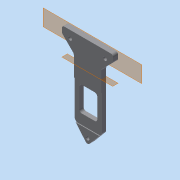
# Autodesk Inventor part: cellSTORM_inverted_chiptray_v0
Saved by Autodesk Inventor 2019.4 (Build 234330000, 330)
## iProperties
Created: 2020-11-09
Part Number: cellSTORM_inverted_chiptray_v0
Material: Generic
Document SubType Name: Modeling
Designer: diederichbenedict
Density: 1 g/cm^3
Appearance: Default
Author: diederichbenedict
Autodesk Inventor part; units mm, degrees
ref_plane "YZ Plane" through (0, 0, 0) normal (1, 0, 0) x (0, 1, 0)
ref_plane "XZ Plane" through (0, 0, 0) normal (0, 1, 0) x (-1, 0, 0)
ref_plane "XY Plane" through (0, 0, 0) normal (0, 0, 1) x (1, 0, 0)
ref_plane "Work Plane1" through (0, 0, 0) normal (0, 0, 1) x (1, 0, 0)
sketch "Sketch1" plane through (0, 0, 0) normal (0, 0, 1) x (1, 0, 0)
  circle A0 centre (-18, 0) radius 2.45 construction
  circle A1 centre (-32.0354, 0) radius 2.45 construction
  circle A2 centre (-48, 0) radius 3.05 construction
  line L0 (18, 6) -> (-54, 6) construction
  line L1 (-54, -6) -> (-54, 6) construction
  line L2 (-54, -6) -> (18, -6) construction
  line L3 (18, -6) -> (18, 6) construction
  circle A3 centre (12, 0) radius 3.05 construction
  circle A4 centre (-3.9646, 0) radius 2.45 construction
  circle A5 centre (-18, -62.5107) radius 2.45 construction
  circle A6 centre (-3.9646, -62.1646) radius 2.45 construction
  circle A7 centre (12, -70) radius 3.05 construction
  line L4 (-32.0354, -67.7344) -> (-3.9646, -67.7344) construction
  line L5 (-3.9646, -67.7344) -> (14.2856, -76.6915) construction
  line L6 (14.2856, -76.6915) -> (18.6915, -67.7144) construction
  line L7 (18.6915, -67.7144) -> (-2.5545, -57.2869) construction
  line L8 (-33.4455, -57.2869) -> (-2.5545, -57.2869) construction
  line L9 (-54.6915, -67.7144) -> (-33.4455, -57.2869) construction
  line L10 (-50.2856, -76.6915) -> (-54.6915, -67.7144) construction
  line L11 (-32.0354, -67.7344) -> (-50.2856, -76.6915) construction
  circle A8 centre (-48, -70) radius 3.05 construction
  circle A9 centre (-32.0354, -62.1646) radius 2.45 construction
  line L12 (-30, -24.7225) -> (-6, -24.7225) construction
  line L13 (-6, -24.7225) -> (-6, -18.4525) construction
  line L14 (-6, -18.4525) -> (-30, -18.4525) construction
  line L15 (-30, -18.4525) -> (-30, -24.7225) construction
  line L16 (-6, -33.7225) -> (-11.7463, -33.7225) construction
  line L17 (-6, -33.34) -> (-6, -33.7225) construction
  line L18 (-6, -33.34) -> (-11.7042, -33.34) construction
  line L19 (-6, -32.95) -> (-6, -33.34) construction
  line L20 (-6, -32.95) -> (-11.6853, -32.95) construction
  line L21 (-6, -32.56) -> (-6, -32.95) construction
  line L22 (-6, -32.56) -> (-11.6906, -32.56) construction
  line L23 (-6, -32.17) -> (-6, -32.56) construction
  line L24 (-6, -32.17) -> (-11.72, -32.17) construction
  line L25 (-6, -31.78) -> (-6, -32.17) construction
  line L26 (-6, -31.78) -> (-11.7739, -31.78) construction
  line L27 (-6, -31.39) -> (-6, -31.78) construction
  line L28 (-6, -31.39) -> (-11.8531, -31.39) construction
  line L29 (-6, -31) -> (-6, -31.39) construction
  line L30 (-6, -31) -> (-11.9583, -31) construction
  line L31 (-6, -30.61) -> (-6, -31) construction
  line L32 (-6, -30.61) -> (-12.0912, -30.61) construction
  line L33 (-6, -30.22) -> (-6, -30.61) construction
  line L34 (-6, -30.22) -> (-12.2534, -30.22) construction
  line L35 (-6, -29.83) -> (-6, -30.22) construction
  line L36 (-6, -29.83) -> (-12.4478, -29.83) construction
  line L37 (-6, -29.44) -> (-6, -29.83) construction
  line L38 (-6, -29.44) -> (-12.6777, -29.44) construction
  line L39 (-6, -29.05) -> (-6, -29.44) construction
  line L40 (-6, -29.05) -> (-12.948, -29.05) construction
  line L41 (-6, -28.66) -> (-6, -29.05) construction
  line L42 (-6, -28.66) -> (-13.2656, -28.66) construction
  line L43 (-6, -24.7225) -> (-6, -28.66) construction
  line L44 (-30, -24.7225) -> (-6, -24.7225) construction
  line L45 (-30, -28.66) -> (-30, -24.7225) construction
  line L46 (-22.7344, -28.66) -> (-30, -28.66) construction
  line L47 (-30, -29.05) -> (-30, -28.66) construction
  line L48 (-23.052, -29.05) -> (-30, -29.05) construction
  line L49 (-30, -29.44) -> (-30, -29.05) construction
  line L50 (-23.3223, -29.44) -> (-30, -29.44) construction
  line L51 (-30, -29.83) -> (-30, -29.44) construction
  line L52 (-23.5522, -29.83) -> (-30, -29.83) construction
  line L53 (-30, -30.22) -> (-30, -29.83) construction
  line L54 (-23.7466, -30.22) -> (-30, -30.22) construction
  line L55 (-30, -30.61) -> (-30, -30.22) construction
  line L56 (-23.9088, -30.61) -> (-30, -30.61) construction
  line L57 (-30, -31) -> (-30, -30.61) construction
  line L58 (-24.0417, -31) -> (-30, -31) construction
  line L59 (-30, -31.39) -> (-30, -31) construction
  line L60 (-24.1469, -31.39) -> (-30, -31.39) construction
  line L61 (-30, -31.78) -> (-30, -31.39) construction
  line L62 (-24.2261, -31.78) -> (-30, -31.78) construction
  line L63 (-30, -32.17) -> (-30, -31.78) construction
  line L64 (-24.28, -32.17) -> (-30, -32.17) construction
  line L65 (-30, -32.56) -> (-30, -32.17) construction
  line L66 (-24.3094, -32.56) -> (-30, -32.56) construction
  line L67 (-30, -32.95) -> (-30, -32.56) construction
  line L68 (-24.3147, -32.95) -> (-30, -32.95) construction
  line L69 (-30, -33.34) -> (-30, -32.95) construction
  line L70 (-24.2958, -33.34) -> (-30, -33.34) construction
  line L71 (-30, -33.7225) -> (-30, -33.34) construction
  line L72 (-24.2537, -33.7225) -> (-30, -33.7225) construction
  line L73 (-7.4129, -57.0165) -> (-7.4129, -24.5897) construction
  line L74 (-21.9151, -37.7958) -> (-30, -37.7958) construction
  line L75 (-30, -37.7958) -> (-30, -44.4525) construction
  line L76 (-30, -44.4525) -> (-6, -44.4525) construction
  line L77 (-6, -44.4525) -> (-6, -37.7958) construction
  line L78 (-6, -37.7958) -> (-14.0849, -37.7958) construction
  line L79 (-29, -9.8284) -> (-29, -53.5585)
  line L80 (-7, -53.5585) -> (-7, -9.8284)
  line L81 (-7.4685, -54.8448) -> (-16.4685, -65.5601)
  line L82 (-19.5315, -65.5601) -> (-28.5315, -54.8448)
  line L83 (-6.4142, -8.4142) -> (2, 0)
  line L84 (-7, -9) -> (4.8995, -9) construction
  line L85 (2.5858, 1.4142) -> (2.5858, 4)
  line L86 (-29.5858, -8.4142) -> (-38, 0)
  line L87 (-29, -9) -> (-17.1005, -9) construction
  line L88 (-38.5858, 1.4142) -> (-38.5858, 4)
  line L89 (0.5858, 6) -> (-36.5858, 6)
  circle A10 centre (-3.9646, 0) radius 1.45
  circle A11 centre (-32.0354, 0) radius 1.45
  circle A12 centre (-18, -62.5107) radius 1.45
  arc A13 (-19.5315, -65.5601) -> (-16.4685, -65.5601) centre (-18, -64.2738) ccw
  arc A14 (-7.4685, -54.8448) -> (-7, -53.5585) centre (-9, -53.5585) ccw
  arc A15 (-29, -53.5585) -> (-28.5315, -54.8448) centre (-27, -53.5585) ccw
  arc A16 (-6.4142, -8.4142) -> (-7, -9.8284) centre (-5, -9.8284) ccw
  arc A17 (-29, -9.8284) -> (-29.5858, -8.4142) centre (-31, -9.8284) ccw
  arc A18 (-36.5858, 6) -> (-38.5858, 4) centre (-36.5858, 4) ccw
  arc A19 (2.5858, 4) -> (0.5858, 6) centre (0.5858, 4) ccw
  arc A20 (2, 0) -> (2.5858, 1.4142) centre (0.5858, 1.4142) ccw
  arc A21 (-38.5858, 1.4142) -> (-38, 0) centre (-36.5858, 1.4142) ccw
  arc A22 (-21.9151, -37.7958) -> (-14.0849, -37.7958) centre (-18, -32.8401) ccw projected
  arc A23 (-24.2537, -33.7225) -> (-11.7463, -33.7225) centre (-18, -32.8401) ccw projected
  point P0 (0, 0)
  point P1 (2.5858, 6)
  point P2 (-38.5858, 6)
  dimension "d0" = 1
  dimension "d1" = 1
  dimension "d4" = 45
  dimension "d5" = 135
  dimension "d6" = 2.9
  dimension "d7" = 2.9
  dimension "d8" = 2.9
  dimension "d9" = 2
  constraints: 22 end point, 18 point on circle, 18 tangent, 12 centre point, 10 point on line, 8 equal radius, 3 coincident, 2 equal length, 2 horizontal, 1 collinear, 1 parallel, 1 perpendicular, 1 vertical
  measures "d0" distance between parallel lines of L80 L13
  measures "d1" distance between parallel lines of L15 L79
  measures "d4" angle of L84 L83
  measures "d5" angle of L87 L86
  measures "d6" diameter of A10
  measures "d7" diameter of A11
  measures "d8" diameter of A12
  measures "d9" radius of A13
extrude "Extrusion1" add sketch "Sketch1" along normal blind 4
sketch "Sketch2" plane through (-29, -53.5585, 0) normal (-1, 0, 0) x (0, 0, 1)
  line L0 (-1.5567, 7.7184) -> (-1.5567, 33.7184) projected
  line L1 (4.4433, 27.7184) -> (4.4433, 13.7184) projected
  line L2 (-41.5567, 33.7184) -> (-41.5567, 7.7184) projected
  line L3 (10.4433, 9.1059) -> (10.4433, 35.1059) projected
  line L4 (10.6133, 9.1059) -> (10.6133, 15.7626) projected
  line L5 (4.3679, 25.1128) -> (4.3679, 21.8128) projected
  line L6 (4.3679, 15.0628) -> (4.3679, -1.8872) projected
  line L7 (3.3679, 25.1128) -> (4.3679, 25.1128) projected
  line L8 (3.3679, -1.8872) -> (4.3679, -1.8872) projected
  line L9 (5.9789, -2.5856) -> (3.3679, -2.5856)
  line L10 (3.3679, -2.5856) -> (3.3679, 27.9738)
  line L11 (3.3679, 27.9738) -> (5.9789, 27.9738)
  line L12 (5.9789, 27.9738) -> (5.9789, -2.5856)
  point P0 (0, 53.5585)
  constraints: 8 end point, 2 parallel, 1 horizontal, 1 perpendicular
extrude "Extrusion2" cut sketch "Sketch2" against normal through all
sketch "Sketch3" plane through (-29, -44.6525, 4) normal (0, 0, 1) x (1, 0, 0)
  line L0 (0, 19.0679) -> (22, 19.0679) projected
  line L1 (0.4269, -10.7931) -> (24.1869, -10.7931) projected
  line L2 (5.8029, 16.5283) -> (16.1971, 16.5283)
  line L3 (18.1971, 14.5283) -> (18.1971, -1.4892)
  line L4 (16.1971, -3.4892) -> (5.8029, -3.4892)
  line L5 (3.8029, -1.4892) -> (3.8029, 14.5283)
  line L6 (3.8029, 16.5283) -> (18.1971, -3.4892) construction
  line L7 (18.1971, 16.5283) -> (3.8029, -3.4892) construction
  arc A0 (5.8029, 16.5283) -> (3.8029, 14.5283) centre (5.8029, 14.5283) ccw
  arc A1 (18.1971, 14.5283) -> (16.1971, 16.5283) centre (16.1971, 14.5283) ccw
  arc A2 (16.1971, -3.4892) -> (18.1971, -1.4892) centre (16.1971, -1.4892) ccw
  arc A3 (3.8029, -1.4892) -> (5.8029, -3.4892) centre (5.8029, -1.4892) ccw
  point P0 (11, 6.5196)
  dimension "d30" = 2
  constraints: 12 end point, 8 point on circle, 8 point on line, 8 tangent, 4 centre point, 3 equal radius, 2 midpoint, 2 parallel, 1 horizontal, 1 perpendicular
  measures "d30" radius of A0
extrude "Extrusion3" cut sketch "Sketch3" against normal through all
chamfer "Chamfer1" [suppressed]
ref_plane "Work Plane2" through (-36.5858, -16, 0) normal (0, 1, 0) x (1, 0, 0)
body "Solid1"
